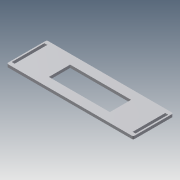
# Autodesk Inventor part: TopFrontPanel
Saved by Autodesk Inventor 2014 (Build 180170000, 170)
## iProperties
Created: 2014-08-11
Part Number: TopFrontPanel
Material: Generic
Document SubType Name: Modeling
Designer: Peele
Density: 1 g/cm^3
Appearance: White
Author: Peele
Autodesk Inventor part; units mm, degrees
ref_plane "YZ Plane" through (0, 0, 0) normal (1, 0, 0) x (0, 1, 0)
ref_plane "XZ Plane" through (0, 0, 0) normal (0, 1, 0) x (-1, 0, 0)
ref_plane "XY Plane" through (0, 0, 0) normal (0, 0, 1) x (1, 0, 0)
sketch "Sketch1" plane through (0, 0, 0) normal (0, 0, 1) x (1, 0, 0)
  line L0 (-134, -42.5) -> (134, -42.5)
  line L1 (134, -42.5) -> (134, 42.5)
  line L2 (134, 42.5) -> (-134, 42.5)
  line L3 (-134, 42.5) -> (-134, -42.5)
  line L4 (-134, -42.5) -> (134, 42.5) construction
  line L5 (134, -42.5) -> (-134, 42.5) construction
  point P0 (0, 0)
  dimension "d0" = 85
  dimension "d1" = 268
  constraints: 12 end point, 2 midpoint, 2 parallel, 1 horizontal, 1 perpendicular
  measures "d0" distance of L2.end L0.start
  measures "d1" distance of L0.start L0.end
extrude "Extrusion1" add sketch "Sketch1" along normal blind 6
sketch "Sketch2" plane through (0, 0, 6) normal (0, 0, 1) x (1, 0, 0)
  line L0 (-134, -42.5) -> (134, -42.5) projected
  line L1 (134, -42.5) -> (134, 42.5) projected
  line L2 (-131.125, -34.5) -> (-124.875, -34.5)
  line L3 (-124.875, -34.5) -> (-124.875, 34.5)
  line L4 (-124.875, 34.5) -> (-131.125, 34.5)
  line L5 (-131.125, 34.5) -> (-131.125, -34.5)
  line L6 (-131.125, -34.5) -> (-124.875, 34.5) construction
  line L7 (-124.875, -34.5) -> (-131.125, 34.5) construction
  line L8 (124.875, -34.5) -> (131.125, -34.5)
  line L9 (131.125, -34.5) -> (131.125, 34.5)
  line L10 (131.125, 34.5) -> (124.875, 34.5)
  line L11 (124.875, 34.5) -> (124.875, -34.5)
  line L12 (124.875, -34.5) -> (131.125, 34.5) construction
  line L13 (131.125, -34.5) -> (124.875, 34.5) construction
  line L14 (134, 42.5) -> (-134, 42.5) projected
  line L15 (-134, 42.5) -> (-134, -42.5) projected
  point P0 (0, 0)
  point P1 (-128, 0)
  point P2 (128, 0)
  dimension "d5" = 2.875
  dimension "d6" = 6.25
  dimension "d8" = 8
  dimension "d34" = 2.875
  dimension "d35" = 8
  constraints: 24 end point, 4 midpoint, 4 parallel, 2 equal length, 2 horizontal, 2 perpendicular, 1 collinear
  measures "d5" distance between parallel lines of L9 L1
  measures "d6" distance of L9.end L10.end
  measures "d8" distance between parallel lines of L2 L0
  measures "d34" distance between parallel lines of L15 L5
  measures "d35" distance between parallel lines of L14 L4
extrude "Extrusion2" cut sketch "Sketch2" against normal through all contours L5 L4 L3 L2 | L11 L10 L9 L8
fillet "Fillet1" radius 3 4 edges at (134, -42.5, 3) (134, 42.5, 3) (-134, -42.5, 3) (-134, 42.5, 3)
sketch "Sketch4" plane through (0, 0, 6) normal (0, 0, 1) x (1, 0, 0)
  line L0 (64.5, -22.5) -> (-64.5, -22.5)
  line L1 (-64.5, -22.5) -> (-64.5, 22.5)
  line L2 (-64.5, 22.5) -> (64.5, 22.5)
  line L3 (64.5, 22.5) -> (64.5, -22.5)
  line L4 (64.5, -22.5) -> (-64.5, 22.5) construction
  line L5 (-64.5, -22.5) -> (64.5, 22.5) construction
  line L6 (131, 42.5) -> (-131, 42.5) projected
  line L7 (-131, -42.5) -> (131, -42.5) projected
  line L8 (0, -42.5) -> (0, 0) construction
  dimension "d2" = 6
  dimension "d33" = 20
  dimension "d36" = 129
  dimension "d37" = 20
  constraints: 14 end point, 3 midpoint, 2 parallel, 1 horizontal, 1 perpendicular, 1 vertical
  measures "d33" distance between parallel lines of L6 L2
  measures "d36" distance of L1.end L2.end
  measures "d37" distance between parallel lines of L7 L0
extrude "Extrusion5" cut sketch "Sketch4" against normal blind 10
equation "\"d34\" = d5"
body "Solid1"
